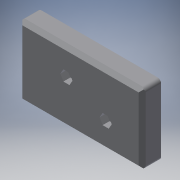
# Autodesk Inventor part: bumper cover upper
Saved by Autodesk Inventor 2019 (Build 230136000, 136)
## iProperties
Created: 2018-12-04
Part Number: bumper cover upper
Material: Generic
Document SubType Name: Modeling
Designer: Varga Daniel
Density: 1 g/cm^3
Appearance: Default
Author: Varga Daniel
Autodesk Inventor part; units mm, degrees
ref_plane "YZ Plane" through (0, 0, 0) normal (1, 0, 0) x (0, 1, 0)
ref_plane "XZ Plane" through (0, 0, 0) normal (0, 1, 0) x (-1, 0, 0)
ref_plane "XY Plane" through (0, 0, 0) normal (0, 0, 1) x (1, 0, 0)
sketch "Sketch1" plane through (0, 0, 0) normal (0, 0, 1) x (1, 0, 0)
  circle A0 centre (-19.3, 2.19) radius 4 construction
  circle A1 centre (20.7, 2.19) radius 4 construction
  circle A2 centre (20.7, -17.81) radius 4 construction
  circle A3 centre (-29.3, 2.19) radius 4 construction
  circle A4 centre (-29.3, -7.81) radius 4 construction
  circle A5 centre (-12.3, -2.81) radius 3.5 construction
  circle A6 centre (10, -13.11) radius 3.5 construction
  line L0 (30.7, 12.19) -> (-39.3, 12.19)
  line L1 (-39.3, 12.19) -> (-39.3, -27.81)
  line L2 (-39.3, -27.81) -> (30.7, -27.81)
  line L3 (30.7, -27.81) -> (30.7, 12.19)
  circle A7 centre (10, -13.11) radius 1.65
  circle A8 centre (-12.3, -2.81) radius 1.65
  line L4 (28.7, 10.19) -> (-37.3, 10.19) projected
  line L5 (28.7, -25.81) -> (28.7, 10.19) projected
  line L6 (-37.3, -25.81) -> (28.7, -25.81) projected
  line L7 (-37.3, 10.19) -> (-37.3, -25.81) projected
  point P0 (0, 0)
  dimension "d0" = 3.3
  dimension "d1" = 3.3
  constraints: 8 end point, 2 centre point, 2 coincident, 2 parallel, 1 horizontal, 1 perpendicular
  measures "d0" diameter of A7
  measures "d1" diameter of A8
extrude "Extrusion1" add sketch "Sketch1" along normal blind 5.51 contours L3 L2 L1 L0 | L5 L6 L7 L4
sketch "Sketch2" plane through (0, 0, 5.51) normal (0, 0, 1) x (1, 0, 0)
  circle A0 centre (-12.3, -2.81) radius 1.65 construction
  circle A1 centre (10, -13.11) radius 1.65 construction
  line L0 (-39.3, 12.19) -> (-39.3, -27.81) construction
  line L1 (-39.3, -27.81) -> (30.7, -27.81) construction
  line L2 (30.7, -27.81) -> (30.7, 12.19) construction
  line L3 (30.7, 12.19) -> (-39.3, 12.19) construction
  line L4 (8.2679, -16.11) -> (6.5359, -13.11)
  line L5 (6.5359, -13.11) -> (8.2679, -10.11)
  line L6 (8.2679, -10.11) -> (11.7321, -10.11)
  line L7 (11.7321, -10.11) -> (13.4641, -13.11)
  line L8 (13.4641, -13.11) -> (11.7321, -16.11)
  line L9 (11.7321, -16.11) -> (8.2679, -16.11)
  line L10 (-14.0321, -5.81) -> (-15.7641, -2.81)
  line L11 (-15.7641, -2.81) -> (-14.0321, 0.19)
  line L12 (-14.0321, 0.19) -> (-10.5679, 0.19)
  line L13 (-10.5679, 0.19) -> (-8.8359, -2.81)
  line L14 (-8.8359, -2.81) -> (-10.5679, -5.81)
  line L15 (-10.5679, -5.81) -> (-14.0321, -5.81)
  point P0 (0, 0)
  dimension "d4" = 6
  dimension "d6" = 6
  constraints: 24 end point, 3 coincident, 2 parallel, 26 other
  measures "d4" distance between parallel lines of L6 L9
  measures "d6" distance between parallel lines of L12 L15
extrude "Extrusion2" cut sketch "Sketch2" against normal blind 4
sketch "Sketch3" plane through (0, 0, 0) normal (0, 0, -1) x (-1, 0, 0)
  circle A0 centre (12.3, -2.81) radius 1.65 projected
  circle A1 centre (-10, -13.11) radius 1.65 projected
  line L0 (39.3, -27.81) -> (39.3, 12.19) projected
  line L1 (39.3, 12.19) -> (-30.7, 12.19) projected
  line L2 (-30.7, 12.19) -> (-30.7, -27.81) projected
  line L3 (-30.7, -27.81) -> (39.3, -27.81) projected
  line L4 (-30.7, -25.81) -> (-30.7, -12.81) construction
  line L5 (21.3, -27.81) -> (-28.7, -27.81) construction
  line L6 (36.3, -24.81) -> (36.3, 9.19)
  line L7 (36.3, 9.19) -> (-27.7, 9.19)
  line L8 (-27.7, 9.19) -> (-27.7, -24.81)
  line L9 (-27.7, -24.81) -> (36.3, -24.81)
  arc A2 (-30.7, -25.81) -> (-28.7, -27.81) centre (-28.7, -25.81) ccw projected
  line L10 (-30.7, -12.81) -> (-19.7, -12.81) projected
  line L11 (-15.7, -16.81) -> (-19.7, -12.81) projected
  line L12 (-15.7, -16.81) -> (-15.7, -24.81) projected
  line L13 (-15.7, -24.81) -> (21.3, -24.81) projected
  line L14 (21.3, -24.81) -> (21.3, -27.81) projected
  circle A3 centre (-20.7, -17.81) radius 2.5 projected
  point P0 (0, 0)
  point P1 (-30.7, -1.81)
  point P2 (33.3, -27.81)
  dimension "d9" = 3
  constraints: 8 end point, 3 other
  measures "d9" distance between parallel lines of L3 L9
extrude "Extrusion3" add sketch "Sketch3" along normal blind 5.29 contours L3 L14 L9 L6 L7 L8 L10 L2 L1 L0 | L3 A2 L2 L10 L8 L9 L14 | L3 L2 A2
sketch "Sketch4" plane through (0, 0, -5.29) normal (0, 0, -1) x (-1, 0, 0)
  line L0 (36.3, -24.81) -> (-27.7, -24.81) construction
  line L1 (-27.7, -24.81) -> (-27.7, 9.19) construction
  line L2 (-27.7, 9.19) -> (36.3, 9.19) construction
  line L3 (36.3, 9.19) -> (36.3, -24.81) construction
  line L4 (39.3, -27.81) -> (39.3, 12.19) construction
  line L5 (39.3, 12.19) -> (-30.7, 12.19) construction
  line L6 (-30.7, 12.19) -> (-30.7, -27.81) construction
  line L7 (-30.7, -27.81) -> (39.3, -27.81) construction
  line L8 (33.3, -27.81) -> (33.3, -24.81) projected
  line L9 (21.3, -24.81) -> (21.3, -27.81) projected
  line L10 (36.3, -24.81) -> (-27.7, -24.81) projected
  line L11 (-30.7, -27.81) -> (39.3, -27.81) projected
  line L12 (-19.7, -1.81) -> (-30.7, -1.81) projected
  line L13 (-30.7, -12.81) -> (-19.7, -12.81) projected
  line L14 (-27.7, -24.81) -> (-27.7, 9.19) projected
  line L15 (-30.7, 12.19) -> (-30.7, -27.81) projected
  point P0 (0, 0)
extrude "Extrusion4" cut sketch "Sketch4" against normal up to surface (5.29 mm away) contours L11 L9 L10 L8
chamfer "Chamfer1" distance 2 angle 45 4 edges at (-4.3, -27.81, 5.51) (-4.3, 12.19, 5.51) (30.7, -7.81, 5.51) (-39.3, -7.81, 5.51)
fillet "Fillet1" radius 2 4 edges at (-39.3, -27.81, -0.89) (30.7, -27.81, -0.89) (-39.3, 12.19, -0.89) (30.7, 12.19, -0.89)
equation "\"d6\" = d4"
body "Solid1"
